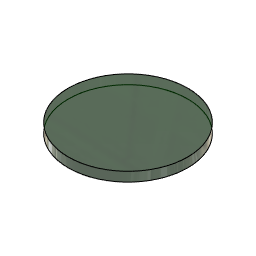
densitometer-dev-cover (Autodesk Fusion 360 archive; units mm, degrees)
design "UV-IR Cut Filter"
Autodesk Fusion 360 part; units mm, degrees
sketch "Sketch1" plane through (0, 0, 0) normal (0, 0, 1) x (1, 0, 0)
  circle A0 centre (0, 0) radius 7
  dimension "d1" = 14
  constraint coincident A0.centre origin
  measures "d1" diameter of A0
extrude "Extrude1" add sketch "Sketch1" along normal blind 1.1

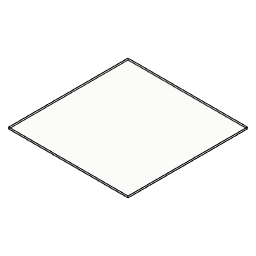
design "Diffuser Material"
Autodesk Fusion 360 part; units mm, degrees
sketch "Sketch1" plane through (0, 0, 0) normal (0, 0, 1) x (1, 0, 0)
  line L0 (7.5, 7.5) -> (-7.5, 7.5)
  line L1 (-7.5, 7.5) -> (-7.5, -7.5)
  line L2 (-7.5, -7.5) -> (7.5, -7.5)
  line L3 (7.5, -7.5) -> (7.5, 7.5)
  line L4 (7.5, 7.5) -> (-7.5, -7.5) construction
  line L5 (-7.5, 7.5) -> (7.5, -7.5) construction
  dimension "d2" = 15
  constraint horizontal L0
  constraint perpendicular L0 L1
  constraint parallel L0 L2
  constraint parallel L1 L3
  constraint coincident L4 origin
  constraint coincident L5 origin
  constraint equal L2 L3
  measures "d2" distance of L0.end L1.end
extrude "Extrude1" add sketch "Sketch1" along normal blind 0.2

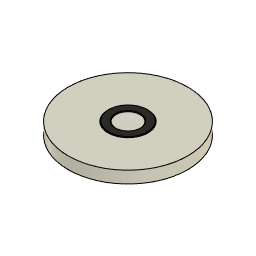
design "Stage Plate"
Autodesk Fusion 360 part; units mm, degrees
sketch "Sketch1" plane through (0, 0, 0) normal (0, 0, 1) x (1, 0, 0)
  circle A0 centre (0, 0) radius 1.5 construction
  circle A1 centre (0, 0) radius 3.2 construction
  circle A2 centre (0, 0) radius 6.2 construction
  circle A3 centre (0, 0) radius 18 construction
  dimension "d1" = 3
  dimension "d2" = 6.4
  dimension "d3" = 12.4
  dimension "d4" = 36
  constraint coincident A0.centre A1.centre
  constraint concentric A0 A1
  constraint concentric A1 A3
  measures "d1" diameter of A0
  measures "d2" diameter of A1
  measures "d3" diameter of A2
  measures "d4" diameter of A3
sketch "Sketch1 (2)" plane through (0, 0, 0) normal (0, 0, 1) x (1, 0, 0) in component "Inner Disc"
  circle A0 centre (0, 0) radius 3
  dimension "d5" = 6
  constraint coincident A0.centre origin
  measures "d5" diameter of A0
extrude "Extrude1" add sketch "Sketch1 (2)" along normal blind 3 makes body 1 in component "Inner Disc"
sketch "Sketch1 (3)" plane through (0, 0, 0) normal (0, 0, 1) x (1, 0, 0) in component "Spacer Ring"
  circle A0 centre (0, 0) radius 3
  circle A1 centre (0, 0) radius 5
  dimension "d8" = 6
  dimension "d9" = 10
  constraint coincident A0.centre A1.centre
  measures "d8" diameter of A0
  measures "d9" diameter of A1
extrude "Extrude1'" add sketch "Sketch1 (3)" along normal blind 3.15 separate body makes body 2 in component "Spacer Ring"
sketch "Sketch1 (4)" plane through (0, 0, 0) normal (0, 0, 1) x (1, 0, 0) in component "Outer Ring"
  circle A0 centre (0, 0) radius 5
  circle A1 centre (0, 0) radius 15
  dimension "d12" = 10
  dimension "d13" = 30
  constraint coincident A0.centre A1.centre
  measures "d12" diameter of A0
  measures "d13" diameter of A1
extrude "Extrude1''" add sketch "Sketch1 (4)" along normal blind 3 separate body makes body 3 in component "Outer Ring"
fillet "Fillet1" radius 0.15 1 edges at (-4.6616, -1.8081, 3.15) on bodies 2 in component "Spacer Ring"
fillet "Fillet2" radius 0.15 1 edges at (-2.797, 1.0848, 3.15) on bodies 2 in component "Spacer Ring"
component "Outer Ring" placed x (1, 0, 0) y (0, 1, 0) z (0, 0, 1) at (0, 0, 0)
component "Spacer Ring" placed x (1, 0, 0) y (0, 1, 0) z (0, 0, 1) at (0, 0, 0)
component "Inner Disc" placed x (1, 0, 0) y (0, 1, 0) z (0, 0, 1) at (0, 0, 0)
